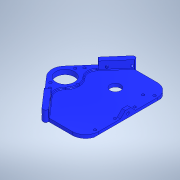
# Autodesk Inventor part: Motor Mount
Saved by Autodesk Inventor 2022 (Build 260153000, 153)
## iProperties
Created: 2022-08-10
Part Number: Motor Mount
Material: Generic
Document SubType Name: Modeling
Designer: Nick
Density: 0.799705 g/cm^3
Appearance: Blue - Wall Paint - Glossy
Mass: 50.56 g
Surface Area: 288.065 cm^2
Volume: 63.2233 cm^3
Author: Nick
Autodesk Inventor part; units mm, degrees
ref_plane "YZ Plane" through (0, 0, 0) normal (1, 0, 0) x (0, 1, 0)
ref_plane "XZ Plane" through (0, 0, 0) normal (0, 1, 0) x (-1, 0, 0)
ref_plane "XY Plane" through (0, 0, 0) normal (0, 0, 1) x (1, 0, 0)
sketch "Sketch14" plane through (0, 0, 0) normal (0, 0, 1) x (1, 0, 0)
  line L0 (0, 0) -> (55, 0)
  line L1 (55, 0) -> (55, 45)
  line L2 (55, 45) -> (0, 45)
  line L3 (0, 45) -> (0, 0)
  circle A0 centre (27.5, 22.5) radius 12.25
  point P0 (55, 22.5)
  point P1 (27.5, 45)
  dimension "d94" = 24.5
  dimension "d95" = 55
  dimension "d96" = 45
  constraints: 8 end point, 2 midpoint, 2 parallel, 1 centre point, 1 horizontal, 1 horizontal alignment, 1 perpendicular, 1 vertical alignment
  measures "d94" diameter of A0
  measures "d95" distance of L0.start L0.end
  measures "d96" distance of L2.end L0.start
extrude "Extrusion13" add sketch "Sketch14" along normal blind 11.26
sketch "Sketch15" plane through (0, 0, 0) normal (0, -1, 0) x (1, 0, 0)
  line L0 (0, 0) -> (55, 0) projected
  line L1 (55, 0) -> (55, 11.26) projected
  line L2 (0, 11.26) -> (55, 11.26) projected
  line L3 (0, 0) -> (0, 11.26) projected
  line L4 (55, 0) -> (55, 11.26) projected
  line L5 (55, 11.26) -> (0, 11.26)
  line L6 (0, 11.26) -> (0, 76.185)
  line L7 (0, 76.185) -> (55, 76.185)
  line L8 (55, 76.185) -> (55, 11.26)
  line L9 (0, 0) -> (0, 11.26) projected
  point P0 (0, 11.26)
  dimension "d99" = 64.925
  constraints: 8 end point, 2 parallel, 1 collinear, 1 horizontal, 1 perpendicular
  measures "d99" distance of L7.end L1.end
extrude "Extrusion14" add sketch "Sketch15" against normal blind 5 contours L6 L7 L8 L2
mirror "Mirror4" about plane through (0, 0, 76.185) normal (0, 0, 1)
sketch "Sketch26" plane through (0, 0, 0) normal (0, -1, 0) x (1, 0, 0)
  line L0 (0, 0) -> (55, 0) projected
  line L1 (0, 0) -> (-55.0618, 63.0266)
  line L2 (0, 152.37) -> (-55.0618, 89.3434)
  arc A0 (-55.0618, 89.3434) -> (-55.0618, 63.0266) centre (-40, 76.185) ccw
  line L3 (0, 0) -> (0, 152.37) projected
  line L4 (0, 0) -> (0, 152.37)
  circle A1 centre (-40, 76.185) radius 14
  point P0 (0, 44.2511)
  point P1 (0, 44.2511)
  dimension "d137" = 20
  dimension "d138" = 40
  dimension "d146" = 28
  constraints: 6 end point, 2 centre point, 2 point on circle, 2 tangent, 1 coincident, 1 equal length, 1 vertical
  measures "d137" radius of A0
  measures "d138" distance from line of L3 A0.centre
  measures "d146" diameter of A1
extrude "Extrusion25" add sketch "Sketch26" against normal blind 5
sketch "Sketch27" plane through (0, 5, 0) normal (0, 1, 0) x (1, 0, 0)
  arc A0 (-55.0618, -63.0266) -> (-55.0618, -89.3434) centre (-40, -76.185) ccw projected
  circle A1 centre (-40, -76.185) radius 14
  circle A2 centre (-40, -76.185) radius 20
  line L0 (0, 0) -> (-55.0618, -63.0266) projected
  line L1 (-55.0618, -89.3434) -> (0, -152.37) projected
  line L2 (55, -141.11) -> (0, -141.11) projected
  line L3 (-26.5102, -110.765) -> (0, -141.11)
  line L4 (0, -11.26) -> (-26.5102, -41.605)
  arc A3 (-26.5102, -41.605) -> (-25.8365, -62.0643) centre (-15.2138, -51.4737) ccw
  arc A4 (-25.8365, -90.3057) -> (-26.5102, -110.765) centre (-15.2138, -100.8963) ccw
  line L5 (-55.0618, -63.0266) -> (0, 0) projected
  line L6 (0, 0) -> (0, -11.26)
  line L7 (0, -141.11) -> (55, -141.11) projected
  line L8 (0, -152.37) -> (0, -141.11) projected
  line L9 (0, -141.11) -> (0, -152.37)
  point P0 (-32.2708, -36.9389)
  point P1 (-29.1283, -59.3979)
  point P2 (-29.1283, -92.9721)
  point P3 (-32.2708, -115.4311)
  point P4 (3, -141.11)
  point P5 (12, -141.11)
  point P6 (-55.0618, -63.0266)
  point P7 (52, -141.11)
  point P8 (51, -141.11)
  dimension "d141" = 28
  dimension "d145" = 15
  constraints: 9 point on circle, 8 end point, 4 centre point, 4 tangent, 2 coincident, 2 parallel, 2 point on line, 1 collinear, 1 equal radius, 1 vertical
  measures "d141" diameter of A1
  measures "d145" radius of A3
extrude "Extrusion26" add sketch "Sketch27" along normal blind 2
sketch "Sketch29" plane through (0, 5, 0) normal (0, 1, 0) x (1, 0, 0)
  circle A0 centre (10, -50.26) radius 14
  circle A1 centre (10, -50.26) radius 8
  line L0 (55, -11.26) -> (0, -11.26) projected
  line L1 (55, -11.26) -> (55, -141.11) projected
  point P0 (0, 0)
  dimension "d149" = 28
  dimension "d151" = 16
  dimension "d202" = 39
  dimension "d203" = 45
  constraints: 2 centre point, 1 coincident
  measures "d149" diameter of A0
  measures "d151" diameter of A1
  measures "d202" distance from line of L0 A0.centre
  measures "d203" distance from line of L1 A0.centre
extrude "Extrusion28" cut sketch "Sketch29" against normal blind 10 contours A1
sketch "Sketch37" plane through (0, 5, 0) normal (0, 1, 0) x (1, 0, 0)
  circle A0 centre (10, -50.26) radius 8 projected
  line L0 (-26.5102, -110.765) -> (0, -141.11) projected
  line L1 (0, -141.11) -> (55, -141.11) projected
  line L2 (55, -11.26) -> (55, -141.11) projected
  line L3 (0, -11.26) -> (55, -11.26) projected
  line L4 (0, -11.26) -> (-26.5102, -41.605) projected
  arc A1 (-26.5102, -41.605) -> (-25.8365, -62.0643) centre (-15.2138, -51.4737) ccw projected
  arc A2 (-25.8365, -90.3057) -> (-25.8365, -62.0643) centre (-40, -76.185) ccw projected
  arc A3 (-25.8365, -90.3057) -> (-26.5102, -110.765) centre (-15.2138, -100.8963) ccw projected
  line L5 (0, -141.11) -> (-26.5102, -110.765) projected
  line L6 (0, -152.37) -> (0, -141.11) projected
  line L7 (0, -141.11) -> (0, -152.37)
  line L8 (55, 0) -> (0, 0) projected
  line L9 (0, -11.26) -> (0, 0)
  line L10 (0, -152.37) -> (55, -152.37) projected
  line L11 (55, 0) -> (55, -11.26) projected
  line L12 (0, -152.37) -> (55, -152.37)
  line L13 (55, -152.37) -> (55, 0)
  line L14 (55, 0) -> (0, 0)
  line L15 (0, 0) -> (0, -152.37)
  point P0 (0, -50.26)
  point P1 (0, -40.2475)
  point P2 (0, -141.11)
  constraints: 12 end point, 3 equal length, 1 horizontal, 1 perpendicular, 1 vertical
extrude "Extrusion35" cut sketch "Sketch37" along normal through all contours L1 L13 L10 L6 | L9 L8 L11 L3
sketch "Sketch40" plane through (0, 5, 0) normal (0, 1, 0) x (1, 0, 0)
  line L0 (0, 0) -> (55, 0) projected
  line L1 (55, 0) -> (0, 0)
  line L2 (0, 0) -> (0, -12)
  line L3 (0, -12) -> (55, -12)
  line L4 (55, -12) -> (55, 0)
  line L5 (55, -152.37) -> (55, 0) projected
  line L6 (55, -152.37) -> (0, -152.37)
  line L7 (0, -152.37) -> (0, -140.37)
  line L8 (0, -140.37) -> (55, -140.37)
  line L9 (55, -140.37) -> (55, -152.37)
  line L10 (55, -152.37) -> (0, -152.37) projected
  dimension "d198" = 12
  dimension "d199" = 12
  constraints: 16 end point, 4 parallel, 2 horizontal, 2 perpendicular, 2 point on line
  measures "d198" distance of L2.end L1.end
  measures "d199" distance of L6.end L7.end
extrude "Extrusion38" cut sketch "Sketch40" against normal through all
sketch "Sketch41" plane through (0, 7, 0) normal (0, 1, 0) x (1, 0, 0)
  arc A0 (-25.8365, -90.3057) -> (-25.8365, -62.0643) centre (-40, -76.185) ccw projected
  arc A1 (-26.5102, -41.605) -> (-25.8365, -62.0643) centre (-15.2138, -51.4737) ccw projected
  line L0 (-26.5102, -41.605) -> (0, -11.26) projected
  line L1 (0, 0) -> (0, -11.26) projected
  line L2 (0, 0) -> (-55.0618, -63.0266) projected
  arc A2 (-55.0618, -63.0266) -> (-55.0618, -89.3434) centre (-40, -76.185) ccw projected
  line L3 (-55.0618, -89.3434) -> (0, -152.37) projected
  line L4 (0, -141.11) -> (0, -152.37) projected
  line L5 (0, -141.11) -> (-26.5102, -110.765) projected
  arc A3 (-25.8365, -90.3057) -> (-26.5102, -110.765) centre (-15.2138, -100.8963) ccw projected
  circle A4 centre (-40, -76.185) radius 14 projected
  line L6 (-26.5102, -41.605) -> (0, -11.26) projected
  line L7 (-25.3432, -40.2691) -> (-30.9222, -35.3952)
  line L8 (-25.3432, -112.1009) -> (-30.9222, -116.9748)
  dimension "d204" = 47
  dimension "d205" = 47
  constraints: 4 end point, 4 point on line, 2 perpendicular
  measures "d204" distance from line of point (0, 0) L7
  measures "d205" distance of L3.end L8.end
extrude "Extrusion39" add sketch "Sketch41" along normal blind 10 contours L5 L4 L3 L8 | L7 L2 L1 L0
sketch "Sketch42" plane through (0, 5, 0) normal (0, 1, 0) x (1, 0, 0)
  circle A0 centre (14.5983, -38.97) radius 1.8 projected
  circle A1 centre (14.5983, -113.37) radius 1.8 projected
  circle A2 centre (40.4017, -113.37) radius 1.8 projected
  circle A3 centre (40.4017, -38.97) radius 1.8 projected
  point P0 (0, 0)
hole "Hole5" at (14.5983, 5, 38.97) at (40.4017, 5, 38.97) at (40.4017, 5, 113.37) at (14.5983, 5, 113.37) direction (0, -1, 0) diameter 4 end through all
fillet "Fillet3" radius 4 6 edges at (0, 2.5, 0) (0, 6, 0) (0, 12, 0) (0, 2.5, 152.37) (0, 6, 152.37) (0, 12, 152.37)
sketch "Sketch43" plane through (-40, 0, 76.185) normal (0, -1, 0) x (1, 0, 0)
  circle A0 centre (-3.6237, -18.6812) radius 1.8 projected
  circle A1 centre (19, -0.03) radius 1.8 projected
  circle A2 centre (-3.6237, 18.6212) radius 1.8 projected
  circle A3 centre (3.0578, -26.3292) radius 1.8 projected
  circle A4 centre (33.322, 60.9113) radius 1.8 projected
  circle A5 centre (18.1899, -43.6503) radius 1.8 projected
  circle A6 centre (18.1899, 43.5903) radius 1.8 projected
  circle A7 centre (3.0578, 26.2692) radius 1.8 projected
  circle A8 centre (33.322, -60.9713) radius 1.8 projected
  circle A9 centre (90, 44.97) radius 1.8 projected
  circle A10 centre (90, -45.03) radius 1.8 projected
  circle A11 centre (90, -15.03) radius 1.8 projected
  circle A12 centre (90, 14.97) radius 1.8 projected
  point P0 (40, -76.185)
  point P1 (-3.6237, -18.6812)
  point P2 (3.0578, -26.3292)
  point P3 (19, -0.03)
  point P4 (18.1899, 43.5903)
  point P5 (33.322, 60.9113)
  point P6 (18.1899, -43.6503)
  point P7 (33.322, -60.9713)
  point P8 (90, -45.03)
  point P9 (90, -15.03)
  point P10 (90, 14.97)
  point P11 (90, 44.97)
hole "Hole6" at (-36.9422, 0, 49.8558) at (-21.8101, 0, 32.5347) at (-6.678, 0, 15.2137) at (-21, 0, 76.155) at (-43.6237, 0, 57.5038) at (-21.8101, 0, 119.7753) at (-6.678, 0, 137.0963) at (50, 0, 121.155) at (50, 0, 91.155) at (50, 0, 61.155) at (50, 0, 31.155) at (-36.9422, 0, 102.4542) at (-43.6237, 0, 94.8062) direction (0, 1, 0) diameter 4 depth 7 tip angle 118
fillet "Fillet4" radius 1 12 edges at (-21.8676, 7, 84.624) (-25.9267, 7, 111.433) (-30.2057, 7, 100.4026) (-30.2057, 7, 51.9674) (-25.9267, 7, 40.937) (-21.881, 7, 67.7174) (-30.2057, 5, 51.9674) (-13.2551, 5, 26.4325) (-21.881, 5, 67.7174) (-30.2057, 5, 100.4026) (-13.2551, 5, 125.9375) (-21.8676, 5, 84.624)
chamfer "Chamfer3" distance 1 angle 45 8 edges at (-31.0371, 0, 35.5267) (-2.5945, 0, 6.9134) (0, 0, 11.3292) (-60, 0, 76.185) (-31.0371, 0, 116.8433) (-2.5945, 0, 145.4566) (0, 0, 141.0408) (55, 0, 76.185)
sketch "Sketch44" plane through (-30.9222, 7, 116.9748) normal (-0.7530888, 0, 0.6579189) x (0.6579189, 0, 0.7530888)
  ellipse E0 centre (8.7114, 2) end of major axis (8.7114, 3.7) minor radius 1.7 projected
  ellipse E1 centre (35.7114, 2) end of major axis (35.7114, 3.7) minor radius 1.7 projected
  point P0 (-67.7481, -7)
  point P1 (8.7114, 2)
  point P2 (35.7114, 2)
  constraints: 2 other
hole "Hole7" at (-7.427, 9, 143.8686) at (-25.1908, 9, 123.5352) direction (0.7530888, 0, -0.6579189) diameter 4 depth 8 tip angle 118
sketch "Sketch45" plane through (-30.9222, 7, 35.3952) normal (-0.7530888, 0, -0.6579189) x (-0.6579189, 0, 0.7530888)
  ellipse E0 centre (-8.7791, 2) end of major axis (-8.7791, 3.7) minor radius 1.7 projected
  ellipse E1 centre (-35.7791, 2) end of major axis (-35.7791, 3.7) minor radius 1.7 projected
  point P0 (-47, -7)
hole "Hole8" at (-25.1462, 9, 28.7837) at (-7.3824, 9, 8.4503) direction (0.7530888, 0, 0.6579189) diameter 4 depth 8 tip angle 118
sketch "Sketch46" plane through (55, 5, 140.37) normal (1, 0, 0) x (0, 0, -1)
  line L0 (52.785, 0) -> (60.185, 7.4)
  line L1 (60.185, 7.4) -> (68.185, 7.4)
  line L2 (68.185, 7.4) -> (75.585, 0)
  line L3 (128.37, -4) -> (0, -4) projected
  line L4 (128.37, -4) -> (128.37, 0) projected
  line L5 (128.37, 0) -> (0, 0) projected
  line L6 (0, 0) -> (0, -4) projected
  point P0 (140.37, -5)
  point P1 (64.185, 0)
  point P2 (64.185, 7.4)
  dimension "d241" = 7.4
  dimension "d242" = 8
  dimension "d243" = 135
  constraints: 6 end point, 2 midpoint, 2 point on line, 1 horizontal, 1 perpendicular, 1 vertical alignment
  measures "d241" distance between parallel lines of L5 L1
  measures "d242" distance of L0.end L1.end
  measures "d243" angle of L2 L1
extrude "Extrusion40" add sketch "Sketch46" against normal blind 5 contours L0 L1 L2 L5
sketch "Sketch47" plane through (55, 1, 12) normal (1, 0, 0) x (0, 0, -1)
  circle A0 centre (-64.17, 5.5969) radius 1.7018 projected
  point P0 (12, -1)
  point P1 (-64.17, 5.5969)
hole "Hole9" at (55, 6.5969, 76.17) direction (-1, 0, 0) diameter 4 depth 8
fillet "Fillet5" radius 20 2 edges at (55, 3, 140.37) (55, 3, 12)
body "Solid3"
